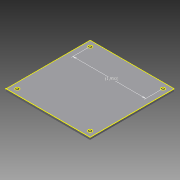
# Autodesk Inventor part: SFE PCB
Saved by Autodesk Inventor 2015 (Build 190159000, 159)
## iProperties
Created: 2016-09-18
Part Number: SFE PCB
Material: Generic
Document SubType Name: Modeling
Designer: spichelh
Density: 1 g/cm^3
Appearance: Default
Author: spichelh
Autodesk Inventor part; units mm, degrees
ref_plane "YZ Plane" through (0, 0, 0) normal (1, 0, 0) x (0, 1, 0)
ref_plane "XZ Plane" through (0, 0, 0) normal (0, 1, 0) x (-1, 0, 0)
ref_plane "XY Plane" through (0, 0, 0) normal (0, 0, 1) x (1, 0, 0)
sketch "Sketch1" plane through (0, 0, 0) normal (0, 1, 0) x (-1, 0, 0)
  line L0 (0, 0) -> (-57.15, 0)
  line L1 (-57.15, 0) -> (-57.15, -57.15)
  line L2 (-57.15, -57.15) -> (0, -57.15)
  line L3 (0, -57.15) -> (0, 0)
  circle A0 centre (-3.81, -3.81) radius 1.27
  line L4 (-28.575, 0) -> (-28.575, -57.15) construction
  line L5 (0, -28.575) -> (-57.15, -28.575) construction
  circle A1 centre (-3.81, -53.34) radius 1.27
  circle A2 centre (-53.34, -3.81) radius 1.27
  circle A3 centre (-53.34, -53.34) radius 1.27
  dimension "d0" = 57.15
  dimension "d1" = 57.15
  dimension "d2" = 3.81
  dimension "d3" = 2.54
  dimension "d4" = 3.81
  constraints: 12 end point, 4 centre point, 4 midpoint, 3 symmetric about line, 2 parallel, 1 horizontal, 1 perpendicular, 3 other
  measures "d0" distance of L2.end L0.start
  measures "d1" distance of L0.start L0.end
  measures "d2" distance from line of L0 A0.centre
  measures "d3" diameter of A0
  measures "d4" distance from line of L3 A0.centre
extrude "Extrusion1" add sketch "Sketch1" along normal blind 1.6
sketch "Sketch2" plane through (0, 1.6, 0) normal (0, 1, 0) x (1, 0, 0)
  circle A0 centre (53.34, 53.34) radius 1.27 projected
  circle A1 centre (53.34, 3.81) radius 1.27 projected
  circle A2 centre (3.81, 53.34) radius 1.27 projected
  circle A3 centre (3.81, 3.81) radius 1.27 projected
  line L0 (0, 0) -> (57.15, 0) projected
  line L1 (57.15, 0) -> (57.15, 57.15) projected
  line L2 (57.15, 57.15) -> (0, 57.15) projected
  line L3 (0, 57.15) -> (0, 0) projected
  dimension "d7" = 49.53
  measures "d7" distance of A0.centre A2.centre
body "Solid1"
